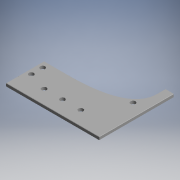
# Autodesk Inventor part: C-head-side
Saved by Autodesk Inventor 2016 (Build 200138000, 138)
## iProperties
Created: 2015-05-08
Part Number: C-head-side
Material: Generic
Document SubType Name: Modeling
Designer: ax
Density: 1 g/cm^3
Appearance: Default
Mass: 3.27214 g
Surface Area: 37.7939 cm^2
Volume: 3.27214 cm^3
Author: ax
Autodesk Inventor part; units mm, degrees
ref_plane "YZ Plane" through (0, 0, 0) normal (1, 0, 0) x (0, 1, 0)
ref_plane "XZ Plane" through (0, 0, 0) normal (0, 1, 0) x (-1, 0, 0)
ref_plane "XY Plane" through (0, 0, 0) normal (0, 0, 1) x (1, 0, 0)
sketch "Sketch1" plane through (0, 0, 0) normal (0, 0, 1) x (1, 0, 0)
  line L0 (0, 0) -> (0, 36)
  line L1 (0, 36) -> (66, 36)
  line L2 (66, 36) -> (66, -7)
  line L3 (66, -7) -> (0, -7)
  line L4 (0, -7) -> (0, 0)
  dimension "d24" = 36
  dimension "d26" = 66
  dimension "d27" = 43
  dimension "d28" = 66
  constraints: 10 end point, 2 perpendicular, 1 point on line, 1 vertical
  measures "d24" distance of L0.start L0.end
  measures "d26" distance of L0.end L1.end
  measures "d27" distance of L1.end L2.end
  measures "d28" distance of L2.end L3.end
extrude "Extrusion1" add sketch "Sketch1" along normal blind 2
sketch "Sketch2" plane through (0, 0, 2) normal (0, 0, 1) x (1, 0, 0)
  line L0 (0, 36) -> (66, 36) projected
  line L1 (0, 36) -> (60, 36)
  line L2 (60, 36) -> (60, 30)
  line L3 (0, 36) -> (0, -7) projected
  line L4 (0, 36) -> (0, 15)
  line L5 (0, 15) -> (16.5, 15)
  line L6 (16.5, 15) -> (60, 15) construction
  line L7 (60, 15) -> (60, 30) construction
  spline S0 degree 2 poles (16.5, 15) (60, 15) (60, 30) knots 1 1 1 2 2 2
  point P0 (0, 0)
  dimension "d29" = 60
  dimension "d30" = 6
  dimension "d31" = 21
  dimension "d33" = 16.5
  constraints: 8 end point, 2 perpendicular, 2 point on line, 1 horizontal, 3 other
  measures "d29" distance of L0.start L1.end
  measures "d30" distance of L1.end L2.end
  measures "d31" distance of L0.start L4.end
  measures "d33" distance of L4.end L5.end
extrude "Extrusion2" cut sketch "Sketch2" against normal through all
chamfer "Chamfer1" distance 0.2 angle 45 9 edges at (49.125, 18.75, 2) (8.25, 15, 2) (60, 33, 2) (66, 14.5, 2) (63, 36, 2) (66, 36, 1) (60, 36, 1) (0, 4, 2) (33, -7, 2)
sketch "Sketch3" plane through (0, 0, 2) normal (0, 0, 1) x (1, 0, 0)
  point P0 (63, 26)
  point P1 (63, 43)
hole "Hole1" at (63, 26, 2) at (63, 43, 2) direction (0, 0, -1) diameter 3.4 depth 2
sketch "Sketch4" plane through (0, 0, 2) normal (0, 0, 1) x (1, 0, 0)
  point P0 (19, 3)
  point P1 (37.5, 3)
  point P2 (56, 3)
hole "Hole3" at (19, 3, 2) at (37.5, 3, 2) at (56, 3, 2) direction (0, 0, -1) diameter 3.4 depth 2
sketch "Sketch5" plane through (0, 0, 0) normal (0, 0, -1) x (-1, 0, 0)
  point P0 (-3, 15.4)
  point P1 (-3, 7.4)
hole "Hole5" at (3, 15.4, 0) at (3, 7.4, 0) direction (0, 0, 1) diameter 3.4 depth 2
equation "\"d24\" = d2 + cMotorSize"
equation "\"d26\" = d0"
equation "\"d28\" = d0"
equation "\"d30\" = d2"
equation "\"d31\" = d2 + 0.5 * cMotorSize"
equation "\"d33\" = 0.25 * d0"
equation "\"d0\" = 66"
equation "\"d2\" = 6"
equation "\"cMotorSize\" = 30"
body "Solid1"
